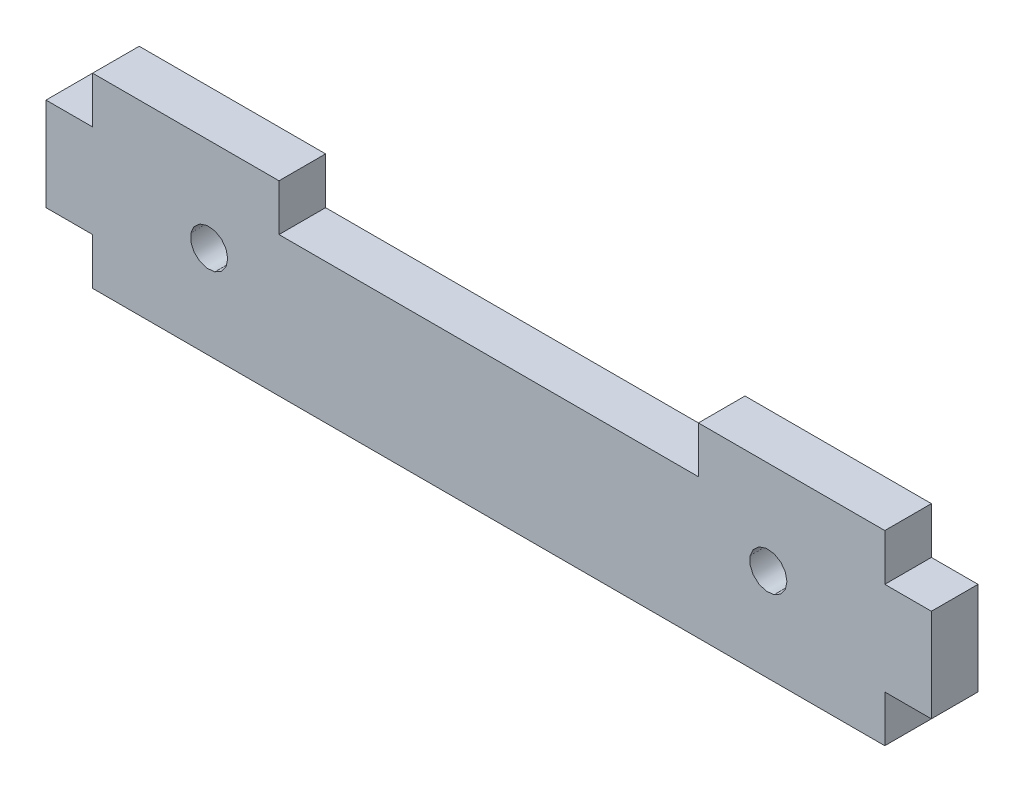
# Autodesk Inventor part: AP
Saved by Autodesk Inventor 2022 (Build 260153000, 153)
## iProperties
Created: 2021-07-09
Part Number: AP
Material: Generic
Document SubType Name: Modeling
Designer: benka
Density: 1 g/cm^3
Appearance: Light Red
Author: benka
Autodesk Inventor part; units mm, degrees
ref_plane "YZ Plane" through (0, 0, 0) normal (1, 0, 0) x (0, 1, 0)
ref_plane "XZ Plane" through (0, 0, 0) normal (0, 1, 0) x (-1, 0, 0)
ref_plane "XY Plane" through (0, 0, 0) normal (0, 0, 1) x (1, 0, 0)
sketch "Sketch1" plane through (0.0001, 0, 0) normal (0, 0, 1) x (1, 0, 0)
  line L0 (47.5003, -5) -> (47.5003, 4.9999)
  line L1 (47.5003, 4.9999) -> (42.5003, 4.9999)
  line L2 (42.5003, 4.9999) -> (42.5003, 9.9999)
  line L3 (42.5003, 9.9999) -> (22.4998, 10)
  line L4 (22.4998, 10) -> (22.4998, 5)
  line L5 (22.4998, 5) -> (-22.5002, 5)
  line L6 (-22.5002, 5) -> (-22.5002, 10)
  line L7 (-22.5002, 10) -> (-42.5005, 10)
  line L8 (-42.5005, 10) -> (-42.5003, 5)
  line L9 (-42.5003, 5) -> (-47.5003, 4.9999)
  line L10 (-47.5003, 4.9999) -> (-47.5, -5)
  line L11 (-47.5, -5) -> (-42.5, -4.9999)
  line L12 (-42.5, -4.9999) -> (-42.4999, -10)
  line L13 (-42.4999, -10) -> (42.5003, -10)
  line L14 (42.5003, -10) -> (42.5003, -5)
  line L15 (42.5003, -5) -> (47.5003, -5)
  circle A0 centre (-30, 0) radius 2
  circle A1 centre (30, 0) radius 2
  point P0 (-0.0005, 0)
  constraints: 32 end point, 2 centre point
extrude "AP" add sketch "Sketch1" along normal blind 5
body "Solid1"
